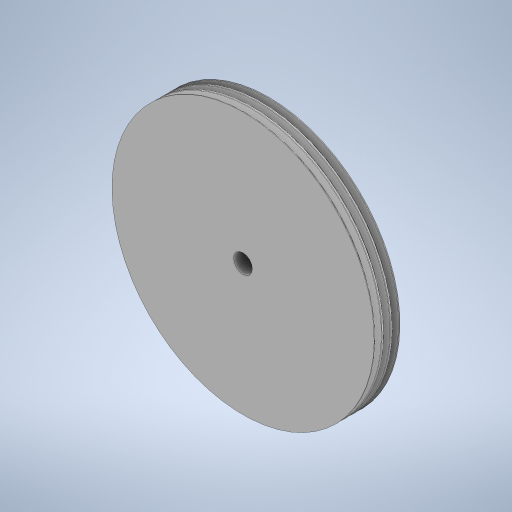
# Autodesk Inventor part: S3-SPS-REMENICE-1
Saved by Autodesk Inventor 2024 (Build 280153000, 153)
## iProperties
Created: 2023-12-19
Part Number: S3-SPS-REMENICE-1
Material: Všeobecné
Document SubType Name: Modeling
Designer: S21Suk
Density: 1 g/cm^3
Appearance: Výchozí
MASSSFP: 400 g
SFP: 4HR
Author: S21Suk
Autodesk Inventor part; units mm, degrees
ref_plane "YZ Plane" through (0, 0, 0) normal (1, 0, 0) x (0, 1, 0)
ref_plane "XZ Plane" through (0, 0, 0) normal (0, 1, 0) x (-1, 0, 0)
ref_plane "XY Plane" through (0, 0, 0) normal (0, 0, 1) x (1, 0, 0)
sketch "Náčrt2" plane through (0, 0, 0) normal (1, 0, 0) x (0, 1, 0)
  line L0 (0, 0) -> (0, -50)
  line L1 (0, 0) -> (250, 0)
  line L2 (250, 0) -> (253.3, 0)
  line L3 (253.3, -50) -> (0, -50)
  line L4 (253.3, 0) -> (253.3, -16.6667)
  line L5 (253.3, -16.6667) -> (253.3, -33.3333)
  line L6 (253.3, -33.3333) -> (253.3, -50)
  line L7 (253.3, -16.6667) -> (0, -16.6667)
  line L8 (253.3, -33.3333) -> (0, -33.3333)
  line L9 (250, 0) -> (241.3, 0)
  line L10 (18, 0) -> (18, -50)
  line L11 (250, 0) -> (250, -50) construction
  line L12 (241.3, 0) -> (241.3, -50)
  line L13 (253.3, -8.3333) -> (241.3, -8.3333)
  line L14 (253.3, -8.3333) -> (253.3, -14.8333) construction
  line L15 (253.3, -14.8333) -> (241.3, -10.9343)
  line L16 (253.3, -1.8333) -> (241.3, -5.7324)
  line L17 (253.3, -18.5) -> (241.3, -22.399)
  line L18 (253.3, -31.5) -> (241.3, -27.601)
  line L19 (253.3, -48.1667) -> (241.3, -44.2676)
  line L20 (253.3, -35.1667) -> (241.3, -39.0657)
  point P0 (241.3, -44.2676)
  dimension "d2" = 50
  dimension "d3" = 250
  dimension "d4" = 3.3
  dimension "d5" = 50
  dimension "d7" = 16.6667
  dimension "d8" = 33.3333
  dimension "d10" = 18
  dimension "d16" = 8.7
  dimension "d19" = 6.5
  dimension "d20" = 18
  constraints: 42 end point, 11 point on line, 10 symmetric about line, 6 perpendicular, 2 horizontal, 2 vertical, 1 collinear, 1 midpoint
  measures "d2" distance of L0.start L0.end
  measures "d3" distance of L0.start L1.end
  measures "d4" distance of L1.end L2.end
  measures "d5" distance of L2.end L3.start
  measures "d7" distance of L4.end L5.end
  measures "d8" diameter of L1 L7
  measures "d10" distance from line of L10 L0.start
  measures "d16" distance between parallel lines of L12 L11
  measures "d19" distance of L13.start L14.end
  measures "d20" angle of L15 L13
revolve "Rotace1" add sketch "Náčrt2" angle 360 about axis through (0, 0, 0) along (0, 0, -1) contours L1 L12 L7 L10 | L7 L12 L8 L10 | L1 L2 L4 L16 L12 | L8 L12 L3 L10 | L12 L15 L4 L7 | L7 L5 L17 L12 | L12 L18 L5 L8 | L8 L6 L20 L12 | L12 L19 L6 L3
fillet "Zaoblení1" radius 1 6 edges at (0, -253.3, -1.8333) (0, -253.3, -14.8333) (0, -253.3, -18.5) (0, -253.3, -35.1667) (0, -253.3, -31.5) (0, -253.3, -48.1667)
